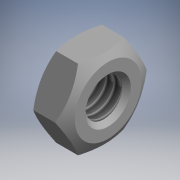
# Autodesk Inventor part: NTJ-010A_CJ2
Saved by Autodesk Inventor 2017.3 (Build 213256000, 256)
## iProperties
Part Number: NTJ-010A_CJ2
Material: Generic
Catalog Web Link: www.cadenas.de
Description: CJ2_NTJ-Rod End Nut
Vendor: SMC
Document SubType Name: Modeling
Designer: partserver
Manufacturer: SMC
Mass: 0.100731 g
Surface Area: 1.58248 cm^2
Volume: 0.100731 cm^3
Density: 1 g/cm^3
Appearance: PSOLRGB-191-191-191
Category: PARTsolutions
Company: SMC
Title: NTJ-010A_CJ2
Author: Cadenas PARTsolutions
Comments: Rod End Nut
PSOL_IDENT_0: {$CADENAS_DATA\23d-libs\smc_jp\actuator\standard_air_cylinder\cj2\accessories\cj2_ntj.prj},165 {VTYP=
PSOL_IDENT_1: 3D},{NB=NTJ-010A_CJ2},{LINA=NTJ-010A_CJ2},{NN=CJ2_NTJ},{DATE=29.10.2021 06:22:45},{GEOMDATE=26.04.20
PSOL_IDENT_2: 20 05:01:36},{VERSION=},{LINEID=20},{WBVAR=},{WBNUMERIC=}  {NB=NTJ-010A_CJ2},{LINA=NTJ-010A_CJ2},{KT=
PSOL_IDENT_3: DUMMY},{MODEL=NTJ-010A},{BORE=10},{B=7.0},{C=8.1},{D=M4x0.7},{D1=4},{D2=0.7},{H=3.2},{DW=5.88},{ORDE
PSOL_IDENT_4: R=NTJ-010A_CJ2}
NB: NTJ-010A_CJ2
NN: CJ2_NTJ
NT: Rod End Nut
NBSYN: $ORDER.
LINA: NTJ-010A_CJ2
CATALOG: SMC (JP
MODEL: NTJ-010A
BORE: 10
B: 7
C: 8.1
D: M4x0.7
H: 3.2
SUPPLIER: SMC
ARTICLENO: NTJ-010A_CJ2
BOMINFO: NTJ-010A_CJ2
CREATOR: CADENAS GmbH
Autodesk Inventor part; units mm, degrees
sketch "B" plane through (0, 0, 0) normal (1, 0, 0) x (0, 1, 0)
  line L0 (-2.0207, 3.5) -> (-4.0415, 0)
  line L1 (-4.0415, 0) -> (-2.0207, -3.5)
  line L2 (-2.0207, -3.5) -> (2.0207, -3.5)
  line L3 (2.0207, -3.5) -> (4.0415, 0)
  line L4 (4.0415, 0) -> (2.0207, 3.5)
  line L5 (2.0207, 3.5) -> (-2.0207, 3.5)
  constraints: 12 end point
extrude "Extrusion1" add sketch "B" along normal mid plane 3.2
sketch "Sketch_2" plane through (0, 0, 0) normal (0, 0, 1) x (1, 0, 0)
  line L0 (1.6, 0) -> (-1.6, 0)
  line L1 (-1.6, 0) -> (-1.6, 2)
  line L2 (-1.6, 2) -> (-1.221, 1.621)
  line L3 (-1.221, 1.621) -> (1.221, 1.621)
  line L4 (1.221, 1.621) -> (1.6, 2)
  line L5 (1.6, 2) -> (1.6, 0)
  line L6 (1.6, 0) -> (-1.6, 0)
  constraints: 14 end point
revolve "Revolution1" cut sketch "Sketch_2" angle 360 about axis through (1.6, 0, 0) along (1, 0, 0)
thread "Thread1" size "M4x0.7" class "6H" standard "ISO Metric profile" full length
sketch "Sketch_3" plane through (0, 0, 0) normal (0, 0, 1) x (1, 0, 0)
  line L0 (50, 0) -> (-50, 0)
  line L1 (-6.6, 6.94) -> (-6.6, 1)
  line L2 (-6.6, 1) -> (-1.6, 1)
  line L3 (-1.6, 1) -> (-1.6, 2.94)
  line L4 (-1.6, 2.94) -> (0, 5.7113)
  line L5 (0, 5.7113) -> (1.6, 2.94)
  line L6 (1.6, 2.94) -> (1.6, 1)
  line L7 (1.6, 1) -> (6.6, 1)
  line L8 (6.6, 1) -> (6.6, 6.94)
  line L9 (6.6, 6.94) -> (-6.6, 6.94)
  constraints: 20 end point
revolve "Revolution2" cut sketch "Sketch_3" angle 360 about axis through (50, 0, 0) along (1, 0, 0)
ref_plane "nt_XY" through (0, 0, 0) normal (1, 0, 0) x (0, 0, -1)
ref_plane "nt_YZ" through (0, 0, 0) normal (0, 0, -1) x (0, 1, 0)
ref_plane "nt_ZX" through (0, 0, 0) normal (0, 1, 0) x (1, 0, 0)
ref_plane "ntj_XY" through (1.6, 0, 0) normal (1, 0, 0) x (0, 0, -1)
ref_plane "ntj_YZ" through (1.6, 0, 0) normal (0, 0, -1) x (0, 1, 0)
ref_plane "ntj_ZX" through (1.6, 0, 0) normal (0, 1, 0) x (1, 0, 0)
body "Solid1"
